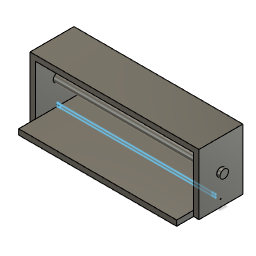
Proto_Derouleur v3 (Autodesk Fusion 360 design; units mm, degrees)
Autodesk Fusion 360 part; units mm, degrees
note: some values were not read from the file. Set by a fixed rule: which face or edge a step refers to.
sketch "Esquisse1" plane through (0, 0, 0) normal (0, 1, 0) x (1, 0, 0)
  line L0 (-250, 65) -> (250, 65)
  line L1 (250, 65) -> (250, -65)
  line L2 (250, -65) -> (-250, -65)
  line L3 (-250, -65) -> (-250, 65)
  line L4 (-250, 65) -> (250, -65) construction
  line L5 (250, 65) -> (-250, -65) construction
  dimension "d1" = 500
  dimension "d2" = 130
  constraint horizontal L0
  constraint perpendicular L0 L1
  constraint parallel L0 L2
  constraint parallel L1 L3
  constraint coincident L4 origin
  constraint coincident L5 origin
  measures "d1" distance of L1.end L2.end
  measures "d2" distance of L0.start L2.end
extrude "Extrusion1" add sketch "Esquisse1" along normal blind 180 makes body 1
shell "Coque1" thickness 16 removed faces 1 at (83.3333, 120, 65) on bodies 1
extrude "Extrusion2" cut 1 faces at (-78, 114.6667, -49) along direction (0, 0, -1) blind 20 on bodies 1 bodies 1
sketch "Esquisse2" plane through (250, 0, 0) normal (1, 0, 0) x (0, 0, -1)
  line L0 (-65, 0) -> (65, 0)
  line L1 (65, 0) -> (65, 180)
  line L2 (65, 180) -> (-65, 180)
  line L3 (-65, 180) -> (-65, 0)
  circle A0 centre (0, 90) radius 12.5
  dimension "d8" = 25
  measures "d8" diameter of A0
extrude "Extrusion3" cut sketch "Esquisse2" against normal blind 3000 contours A0 bodies 1
sketch "Esquisse3" plane through (0, 0, 65) normal (0, 0, 1) x (1, 0, 0)
  line L0 (234, 164) -> (234, 16)
  line L1 (234, 16) -> (-234, 16)
  line L2 (-234, 16) -> (-234, 164)
  line L3 (-234, 164) -> (234, 164)
  line L4 (-250, 0) -> (250, 0)
  line L5 (250, 0) -> (250, 180)
  line L6 (250, 180) -> (-250, 180)
  line L7 (-250, 180) -> (-250, 0)
  line L8 (-250, 16) -> (250, 16)
  line L9 (250, 16) -> (250, 0)
  line L10 (250, 0) -> (-250, 0)
  line L11 (-250, 0) -> (-250, 16)
  constraint horizontal L8
  constraint vertical L9
  constraint horizontal L10
  constraint vertical L11
  constraint coincident L4.end L5.start
  constraint coincident L7 L8.start
extrude "Extrusion4" add sketch "Esquisse3" along normal blind 50 contours L1 L4 L5 L7 L8 L9 L10 L11 bodies 1
sketch "Esquisse4" plane through (250, 0, 0) normal (1, 0, 0) x (0, 0, -1)
  circle A0 centre (0, 90) radius 12.5
  line L0 (-115, 0) -> (65, 0)
  line L1 (65, 0) -> (65, 180)
  line L2 (65, 180) -> (-65, 180)
  line L3 (-65, 180) -> (-65, 16)
  line L4 (-65, 16) -> (-115, 16)
  line L5 (-115, 16) -> (-115, 0)
  circle A1 centre (0, 90) radius 12
  dimension "d13" = 24
  constraint concentric A0 A1
  measures "d13" diameter of A1
extrude "Extrusion5" add sketch "Esquisse4" against normal blind 520 separate body contours A1 makes body 2
sketch "Esquisse5" plane through (250, 0, 0) normal (1, 0, 0) x (0, 0, -1)
  circle A0 centre (0, 90) radius 12.5
  line L0 (-115, 0) -> (65, 0)
  line L1 (65, 0) -> (65, 180)
  line L2 (65, 180) -> (-65, 180)
  line L3 (-65, 180) -> (-65, 16)
  line L4 (-65, 16) -> (-115, 16)
  line L5 (-115, 16) -> (-115, 0)
extrude "Extrusion6" add sketch "Esquisse5" along normal blind 10 contours A0 bodies 2 1
extrude "Extrusion7" cut 1 faces at (-270, 87.222, 5.6039) along direction (1, 0, 0) blind 10 on bodies 2 bodies 2
sketch "Esquisse6" plane through (0, 0, 115) normal (0, 0, 1) x (1, 0, 0)
  line L0 (-250, 0) -> (250, 0)
  line L1 (250, 0) -> (250, 16)
  line L2 (250, 16) -> (-250, 16)
  line L3 (-250, 16) -> (-250, 0)
  line L4 (-250, 16) -> (-234, 16)
  line L5 (-234, 16) -> (-234, 0)
  line L6 (-234, 0) -> (-250, 0)
  line L7 (-250, 0) -> (-250, 16)
  line L8 (250, 0) -> (234, 0)
  line L9 (234, 0) -> (234, 16)
  line L10 (234, 16) -> (250, 16)
  line L11 (250, 16) -> (250, 0)
  dimension "d20" = 16
  dimension "d21" = 16
  dimension "d22" = 16
  dimension "d23" = 16
  constraint horizontal L4
  constraint vertical L5
  constraint horizontal L6
  constraint vertical L7
  constraint coincident L2.end L3.start
  constraint horizontal L8
  constraint vertical L9
  constraint horizontal L10
  constraint vertical L11
  constraint coincident L0.end L1.start
  measures "d20" distance of L2.end L4.end
  measures "d21" distance of L2.end L0.start
  measures "d22" distance of L9.end L1.end
  measures "d23" distance of L8.end L9.end
extrude "Extrusion8" cut sketch "Esquisse6" against normal blind 50 contours L0 L2 L3 L4 L5 L6 L7 | L0 L1 L2 L8 L9 L10 L11 bodies 2
sketch "Esquisse7" plane through (250, 0, 0) normal (1, 0, 0) x (0, 0, -1)
  line L0 (-65, 180) -> (-65, 0)
  line L1 (-65, 0) -> (65, 0)
  line L2 (65, 0) -> (65, 180)
  line L3 (65, 180) -> (-65, 180)
  circle A0 centre (0, 90) radius 12.5
  circle A1 centre (0, 19) radius 1.5
  dimension "d26" = 3
  measures "d26" diameter of A1
extrude "Extrusion9" cut sketch "Esquisse7" against normal blind 9000 contours A1 bodies 2
move_face "DéplacerFace1" to x (1, 0, 0) y (0, 1, 0) z (0, 0, 1) at (0, 1.9859, 0.2369) 1 faces at (-244.6667, 18.9252, 1.4981) on bodies 2
move_face "DéplacerFace2" to x (1, 0, 0) y (0, 1, 0) z (0, 0, 1) at (0, 1.8936, 0.6436) 1 faces at (244.6667, 18.8506, -1.4925) on bodies 2
sketch "Esquisse8" plane through (-250, 0, 0) normal (-1, 0, 0) x (0, 0, 1)
  circle A0 centre (0.2369, 20.9859) radius 1.5
  line L0 (65, 0) -> (65, 180)
  line L1 (65, 180) -> (-65, 180)
  line L2 (-65, 180) -> (-65, 0)
  line L3 (-65, 0) -> (65, 0)
  circle A1 centre (0, 90) radius 12.5
  circle A2 centre (0.2369, 20.9859) radius 1.45
  dimension "d29" = 2.9
  constraint concentric A0 A2
  measures "d29" diameter of A2
extrude "Extrusion10" add sketch "Esquisse8" against normal blind 20 separate body contours A2 makes body 3
sketch "Esquisse9" plane through (250, 0, 0) normal (1, 0, 0) x (0, 0, -1)
  circle A0 centre (-0.6436, 20.8936) radius 1.5
  line L0 (-65, 180) -> (-65, 0)
  line L1 (-65, 0) -> (65, 0)
  line L2 (65, 0) -> (65, 180)
  line L3 (65, 180) -> (-65, 180)
  circle A1 centre (0, 90) radius 12.5
  circle A2 centre (-0.6436, 20.8936) radius 1.45
  dimension "d32" = 2.9
  constraint concentric A0 A2
  measures "d32" diameter of A2
extrude "Extrusion11" add sketch "Esquisse9" against normal blind 20 separate body contours A2 makes body 4
sketch "Esquisse10" plane through (0, 0, 0) normal (0, 0, 1) x (1, 0, 0)
  line L0 (-234, 16) -> (234, 16)
  line L1 (234, 16) -> (234, 25)
  line L2 (234, 25) -> (-234, 25)
  line L3 (-234, 25) -> (-234, 16)
  dimension "d35" = 468
  dimension "d36" = 9
  constraint horizontal L0
  constraint vertical L1
  constraint horizontal L2
  constraint vertical L3
  measures "d35" distance of L1.end L2.end
  measures "d36" distance of L0.end L1.end
sketch "Esquisse11" plane through (0, 0, 0) normal (0, 0, 1) x (1, 0, 0)
  line L0 (-234, 25) -> (-225, 25)
  line L1 (-225, 25) -> (-225, 16)
  line L2 (-225, 16) -> (-234, 16)
  line L3 (-234, 16) -> (-234, 25)
  line L4 (234.0002, 16) -> (225.0002, 16)
  line L5 (225.0002, 16) -> (225.0002, 25)
  line L6 (225.0002, 25) -> (234.0002, 25)
  line L7 (234.0002, 25) -> (234.0002, 16)
  dimension "d37" = 9
  dimension "d38" = 9
  dimension "d39" = 9
  dimension "d40" = 9
  constraint horizontal L0
  constraint vertical L1
  constraint horizontal L2
  constraint vertical L3
  constraint horizontal L4
  constraint vertical L5
  constraint horizontal L6
  constraint vertical L7
  measures "d37" distance of L0.end L1.end
  measures "d38" distance of L0.start L0.end
  measures "d39" distance of L5.end L6.end
  measures "d40" distance of L4.end L5.end
